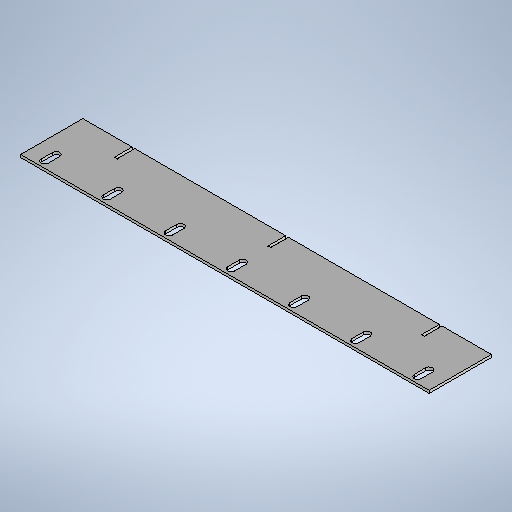
# Autodesk Inventor part: TRM 032 plate
Saved by Autodesk Inventor 2025.1 (Build 291241020, 241B)
## iProperties
Created: 2024-09-08
Part Number: TRM 032 plate
Material: Stainless Steel
Document SubType Name: Sheet Metal
Designer: pokla
Density: 8 g/cm^3
Sheet Metal Rule: AISI304 3mm Die 32
Appearance: Default
Flat Pattern Width: 7 cm
Flat Pattern Length: 46 cm
Flat Pattern Area: 322 cm^2
Sheet Metal Width: 70.000 mm
Sheet Metal Length: 460.000 mm
Sheet Metal Area: 32200.000 mm^2
Author: pokla
Autodesk Inventor part; units mm, degrees
ref_plane "YZ Plane" through (0, 0, 0) normal (1, 0, 0) x (0, 1, 0)
ref_plane "XZ Plane" through (0, 0, 0) normal (0, 1, 0) x (-1, 0, 0)
ref_plane "XY Plane" through (0, 0, 0) normal (0, 0, 1) x (1, 0, 0)
sketch "Sketch1" plane through (0, 0, 0) normal (0, 0, 1) x (1, 0, 0)
  line L0 (-230, 0) -> (230, 0)
  line L1 (230, 0) -> (230, -70)
  line L2 (230, -70) -> (-230, -70)
  line L3 (-230, -70) -> (-230, 0)
  point P0 (0, 0)
  point P1 (0, 0)
  dimension "d0" = 460
  dimension "d1" = 70
  measures "d0" distance of L0.start L0.end
  measures "d1" distance of L2.end L0.start
extrude "Plate1" add sketch "Sketch1" against normal blind 3
sketch "Sketch2" plane through (0, 0, 0) normal (0, 0, 1) x (1, 0, 0)
  line L0 (-230, -70) -> (230, -70) projected
  line L1 (230, -70) -> (230, 0) projected
  line L2 (230, 0) -> (-230, 0) projected
  line L3 (-230, 0) -> (-230, -70) projected
  circle A0 centre (0, -63) radius 4
  circle A1 centre (0, -50) radius 4
  line L4 (4, -63) -> (4, -50)
  line L5 (-4, -63) -> (-4, -50)
  point P0 (0, 0)
  point P1 (0, -70)
  dimension "d3" = 8
  dimension "d5" = 7
  dimension "d22" = 13
  constraints: 4 end point, 4 point on circle, 3 tangent, 2 centre point, 2 vertical alignment, 1 equal radius, 1 midpoint, 1 parallel
  measures "d3" diameter of A0
  measures "d5" distance from line of L0 A0.centre
  measures "d22" distance of A1.centre A0.centre
extrude "Cut1" cut sketch "Sketch2" against normal through all contours A0 | A0 L5 A1 L4 | A1
pattern_linear "Rectangular Pattern1" count 7 spacing 70 along (-1, 0, 0) of "Cut1" first direction both ways yes
sketch "Sketch3" plane through (0, 0, 0) normal (0, 0, 1) x (1, 0, 0)
  line L0 (1.55, -20) -> (-1.55, -20)
  line L1 (-1.55, -20) -> (-1.55, 0)
  line L2 (-1.55, 0) -> (1.55, 0)
  line L3 (1.55, 0) -> (1.55, -20)
  line L4 (230, 0) -> (-230, 0) projected
  point P0 (0, 0)
  point P1 (0, 0)
  point P2 (0, 0)
  dimension "d11" = 3.1
  dimension "d12" = 20
  constraints: 8 end point, 3 midpoint, 2 parallel, 1 horizontal, 1 perpendicular
  measures "d11" distance of L1.end L2.end
  measures "d12" distance of L0.end L1.end
extrude "Cut2" cut sketch "Sketch3" against normal blind 3
pattern_linear "Rectangular Pattern2" count 3 spacing 173 along (-1, 0, 0) of "Cut2" first direction both ways yes
equation "\"d6\" = Thickness"
equation "\"d13\" = Thickness"
equation "\"d2\" = Thickness"
equation "\"BendReliefWidth\" = Thickness"
equation "\"BendReliefDepth\" = 0.5 * Thickness"
equation "\"CornerReliefSize\" = 4 * Thickness"
equation "\"MinimumRemnant\" = 2 * Thickness"
equation "\"TransitionRadius\" = BendRadius"
equation "\"JacobiRadiusSize\" = BendRadius"
equation "\"GapSize\" = Thickness"
equation "\"Thickness\" = 3"
equation "\"BendRadius\" = 5"
body "Solid1"
